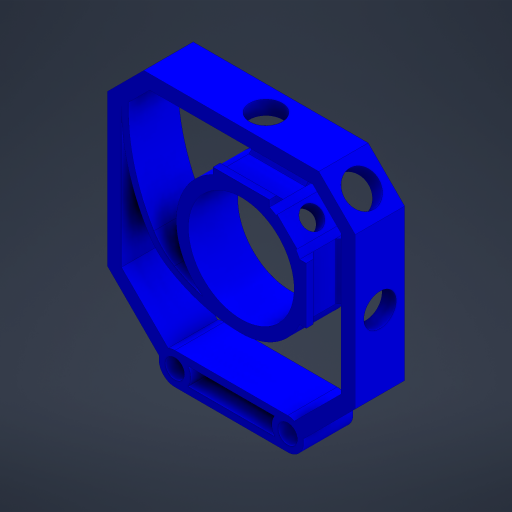
# Autodesk Inventor part: Laser Holder (Green Laser)
Saved by Autodesk Inventor 2023.4 (Build 274418000, 418)
## iProperties
Created: 2022-07-25
Part Number: Laser Holder (Green Laser)
Material: Generic
Document SubType Name: Modeling
Designer: xSibe
Density: 1 g/cm^3
Appearance: Plastic Blue
Author: xSibe
Autodesk Inventor part; units mm, degrees
ref_plane "YZ Plane" through (0, 0, 0) normal (1, 0, 0) x (0, 1, 0)
ref_plane "XZ Plane" through (0, 0, 0) normal (0, 1, 0) x (-1, 0, 0)
ref_plane "XY Plane" through (0, 0, 0) normal (0, 0, 1) x (1, 0, 0)
sketch "Sketch1" plane through (0, 0, 0) normal (0, 0, 1) x (1, 0, 0)
  circle A0 centre (10, 3.85) radius 1.5625
  circle A1 centre (-10, 3.85) radius 1.5625
  line L0 (-16.9, 0) -> (16.9, 0)
  line L1 (16.9, 0) -> (16.9, 7.7)
  line L2 (-16.9, 7.7) -> (16.9, 7.7)
  line L3 (-16.9, 0) -> (-16.9, 7.7)
  circle A2 centre (-10, 3.85) radius 2.8125
  circle A3 centre (10, 3.85) radius 2.8125
  line L4 (-10, 6.6625) -> (10, 6.6625)
  line L5 (10, 1.0375) -> (-10, 1.0375)
  line L6 (-10, 2.2875) -> (10, 2.2875)
  line L7 (-10, 5.4125) -> (10, 5.4125)
  line L8 (-17.05, 7.7) -> (-17.05, 42.1)
  line L9 (17.05, 7.7) -> (17.05, 42.1)
  line L10 (-17.05, 24.9) -> (17.05, 24.9)
  line L11 (0, 24.9) -> (1.767767, 26.667767)
  line L12 (0, 24.9) -> (2.5, 24.9) construction
  circle A4 centre (1.767767, 26.667767) radius 9.375
  circle A5 centre (1.767767, 26.667767) radius 6.875
  circle A6 centre (1.767767, 26.667767) radius 11.5
  line L13 (1.767767, 26.667767) -> (1.767767, 38.167767)
  line L14 (1.767767, 38.167767) -> (1.767767, 37.542767)
  line L15 (-3.232233, 36.917767) -> (6.767767, 36.917767)
  line L16 (6.767767, 36.917767) -> (6.767767, 38.167767)
  line L17 (6.767767, 38.167767) -> (-3.232233, 38.167767)
  line L18 (-3.232233, 38.167767) -> (-3.232233, 36.917767)
  line L19 (-3.232233, 36.917767) -> (6.767767, 38.167767) construction
  line L20 (6.767767, 36.917767) -> (-3.232233, 38.167767) construction
  line L21 (1.767767, 26.667767) -> (9.899495, 34.799495)
  line L22 (9.899495, 34.799495) -> (9.457553, 34.357553)
  line L23 (11.667262, 33.031728) -> (8.131728, 36.567262)
  line L24 (8.131728, 36.567262) -> (7.247845, 35.683378)
  line L25 (7.247845, 35.683378) -> (10.783378, 32.147845)
  line L26 (10.783378, 32.147845) -> (11.667262, 33.031728)
  line L27 (11.667262, 33.031728) -> (7.247845, 35.683378) construction
  line L28 (8.131728, 36.567262) -> (10.783378, 32.147845) construction
  line L29 (11.667262, 33.031728) -> (16.667262, 33.031728) construction
  line L30 (12.017767, 21.667767) -> (12.017767, 31.667767)
  line L31 (12.017767, 31.667767) -> (13.267767, 31.667767)
  line L32 (13.267767, 31.667767) -> (13.267767, 21.667767)
  line L33 (13.267767, 21.667767) -> (12.017767, 21.667767)
  line L34 (1.767767, 38.167767) -> (1.767767, 40.167767)
  line L35 (13.267767, 26.667767) -> (15.267767, 26.667767)
  line L36 (-10.217767, 5.432233) -> (10.217767, 5.432233)
  line L37 (19.467767, 14.682233) -> (19.467767, 39.367767)
  line L38 (14.467767, 44.367767) -> (-14.467767, 44.367767)
  line L39 (-19.467767, 39.367767) -> (-19.467767, 14.682233)
  line L40 (-19.467767, 5.432233) -> (19.467767, 44.367767) construction
  line L41 (19.467767, 5.432233) -> (-19.467767, 44.367767) construction
  line L42 (-10.217767, 5.432233) -> (-19.467767, 14.682233)
  line L43 (10.217767, 5.432233) -> (19.467767, 14.682233)
  line L44 (14.467767, 44.367767) -> (19.467767, 39.367767)
  line L45 (-14.467767, 44.367767) -> (-19.467767, 39.367767)
  line L46 (-15.503301, 46.867767) -> (-21.967767, 40.403301)
  line L47 (-21.967767, 40.403301) -> (-21.967767, 13.646699)
  line L48 (-21.967767, 13.646699) -> (-11.253301, 2.932233)
  line L49 (-11.253301, 2.932233) -> (11.253301, 2.932233)
  line L50 (11.253301, 2.932233) -> (21.967767, 13.646699)
  line L51 (21.967767, 13.646699) -> (21.967767, 40.403301)
  line L52 (21.967767, 40.403301) -> (15.503301, 46.867767)
  line L53 (15.503301, 46.867767) -> (-15.503301, 46.867767)
  circle A7 centre (-10, 3.85) radius 1.705
  circle A8 centre (10, 3.85) radius 1.707
  line L54 (1.767767, 15.167767) -> (-13.232233, 15.167767)
  line L55 (-13.232233, 15.167767) -> (-13.232233, 20.167767)
  arc A9 (-19.467767, 39.367767) -> (-13.232233, 20.167767) centre (13.209618, 39.367767) ccw
  arc A10 (-13.232233, 20.167767) -> (1.767767, 15.167767) centre (1.767767, 40.167767) ccw
  arc A11 (-18.191856, 40.643678) -> (-12.331418, 21.055586) centre (13.209618, 39.367767) ccw
  arc A12 (-12.331418, 21.055586) -> (-5.074449, 17.424711) centre (1.767767, 40.167767) ccw
  line L56 (-12.331418, 21.055586) -> (-13.70616, 23.143667)
  line L57 (-13.232233, 20.167767) -> (-14.62268, 22.245423)
  arc A13 (-13.70616, 23.143667) -> (-10.054119, 19.56909) centre (-4.985941, 28.399978) ccw
  arc A14 (-14.62268, 22.245423) -> (-10.979773, 18.661949) centre (-5.545684, 27.829564) ccw
  point P0 (0, 0)
  point P1 (-7.661464, 2.2875)
  point P2 (-7.661464, 5.4125)
  point P3 (7.661464, 5.4125)
  point P4 (7.661464, 2.2875)
  point P5 (7.341455, 2.932233)
  point P6 (-7.341455, 2.932233)
  point P7 (-11.185824, 6.40029)
  point P8 (11.185824, 6.40029)
  point P9 (-3.232233, 37.023925)
  point P10 (12.123925, 21.667767)
  point P11 (12.123925, 31.667767)
  point P12 (11.472788, 32.837254)
  point P13 (7.937254, 36.372788)
  point P14 (6.767767, 37.023925)
  point P15 (12.751875, 4.430808)
  point P16 (-12.751875, 4.430808)
  dimension "d0" = 1.25
  dimension "d1" = 1.25
  dimension "d2" = 2.5
  dimension "d3" = 45
  dimension "d4" = 18.75
  dimension "d5" = 2.5
  dimension "d6" = 2.125
  dimension "d7" = 0.625
  dimension "d8" = 10
  dimension "d9" = 1.25
  dimension "d10" = 0.625
  dimension "d11" = 5
  dimension "d12" = 135
  dimension "d13" = 1.25
  dimension "d14" = 2
  dimension "d15" = 2
  dimension "d16" = 38.93553
  dimension "d17" = 38.93553
  dimension "d18" = 9.25
  dimension "d19" = 9.25
  dimension "d20" = 9.25
  dimension "d21" = 9.25
  dimension "d22" = 5
  dimension "d23" = 5
  dimension "d24" = 5
  dimension "d25" = 5
  dimension "d26" = 2.5
  dimension "d46" = 0.1425
  dimension "d47" = 0.1445
  dimension "d48" = 15
  dimension "d49" = 5
  dimension "d50" = 1.25
  dimension "d51" = 2.5
  dimension "d52" = 2.5
  constraints: 104 end point, 28 point on circle, 14 tangent, 13 centre point, 12 point on line, 10 midpoint, 8 parallel, 7 horizontal, 7 perpendicular, 4 symmetric about line, 2 equal length, 1 coincident, 1 vertical, 8 other
  measures "d0" radial gap between concentric circles of A1 A2
  measures "d1" radial gap between concentric circles of A0 A3
  measures "d2" distance of L11.start L11.end
  measures "d3" angle of L12 L11
  measures "d4" diameter of A4
  measures "d5" radial gap between concentric circles of A4 A5
  measures "d6" radial gap between concentric circles of A4 A6
  measures "d7" distance of L13.end L14.end
  measures "d8" distance of L17.end L16.end
  measures "d9" distance of L16.end L15.end
  measures "d10" distance of L21.end L22.end
  measures "d11" distance of L23.start L23.end
  measures "d12" angle of L29 L23
  measures "d13" distance of L24.end L23.end
  measures "d14" distance of L13.end L34.end
  measures "d15" distance of L35.start L35.end
  measures "d16" distance of L40.end L41.end
  measures "d17" distance of L41.end L40.start
  measures "d18" distance of L36.start L40.start
  measures "d19" distance of L39.end L40.start
  measures "d20" distance of L36.end L41.start
  measures "d21" distance of L37.start L41.start
  measures "d22" distance of L38.start L40.end
  measures "d23" distance of L37.end L40.end
  measures "d24" distance of L38.end L41.end
  measures "d25" distance of L39.start L41.end
  measures "d26" distance between parallel lines of L38 L53
  measures "d46" radial gap between concentric circles of A1 A7
  measures "d47" radial gap between concentric circles of A0 A8
  measures "d48" distance of L54.start L54.end
  measures "d49" distance of L54.end L55.end
  measures "d50" radial gap between concentric circles of A9 A11
  measures "d51" distance of L56.start L56.end
  measures "d52" distance of L55.end L57.end
extrude "Extrusion1" add sketch "Sketch1" along normal mid plane 8.75 contours A8 L49 A3 L7 | L7 A3 L36 A8 | A8 L43 A3 L50 | L50 A3 L6 A8 | A8 L6 A3 L49 | L7 A2 L36 A3 | L36 A3 L43 A8 | A3 L43 L2 L50 | L36 A2 L4 A3 | L7 A7 L36 A2 | A2 L49 A7 L7 | A3 L5 A2 L6 | L2 L43 L9 L50 | A2 L6 A7 L49 | L36 A7 L42 A2 | A2 L48 A7 L6 | L9 L43 L37 L44 L38 L45 L39 L42 L8 L48 L47 L46 L53 L52 L51 L50 | L42 A2 L48 L2 | L2 L48 L8 L42 | L42 A7 L48 A2 | L32 L33 A6 L10 | L10 A6 L32 | A9 L45 A11 L8 | L8 A11 L10 A9 | L10 A11 A12 A6 A10 A14 L57 A9 | A6 L33 L30 L10 | L10 L30 L31 A6 | A6 L31 L32 | L57 A14 | L30 L33 A6 L10 A4 | L10 A4 L21 L25 L26 A6 L31 L30 | A6 L18 L15 L13 A4 L10 | A13 L56 A11 | L26 L25 L21 A6 | A6 L23 L26 | L18 L17 A6 | A6 L13 L15 L18 | L56 A13 A12 | L21 L25 L24 A6 | A6 L24 L23 | L13 L15 L16 A6 L24 L25 L21 A4 | L17 L16 A6 | A6 L16 L15 L13
sketch "Sketch2" plane through (0, 0, 0) normal (0, 0, 1) x (1, 0, 0)
  circle A0 centre (1.767767, 26.667767) radius 9.375
  circle A1 centre (1.767767, 26.667767) radius 7.5
  point P0 (0, 0)
  dimension "d30" = 1.875
  constraints: 1 centre point
  measures "d30" radial gap between concentric circles of A0 A1
extrude "Extrusion2" [suppressed]
sketch "Sketch3" plane through (21.967767, 13.646699, -4.375) normal (1, 0, 0) x (0, 0, -1)
  line L0 (0, 8.021068) -> (-8.75, 8.021068)
  line L1 (0, 18.021068) -> (0, 8.021068)
  line L2 (0, 18.021068) -> (-8.75, 18.021068)
  line L3 (-8.75, 8.021068) -> (-8.75, 18.021068)
  line L4 (-4.375, 18.021068) -> (-4.375, 8.021068)
  circle A0 centre (-4.375, 13.021068) radius 2.875
  point P0 (-4.375, -13.646699)
  dimension "d33" = 5.75
  constraints: 3 midpoint, 2 end point, 1 centre point
  measures "d33" diameter of A0
extrude "Extrusion3" cut sketch "Sketch3" against normal up to surface (2.5 mm away) contours A0 L4 | L4 A0
sketch "Sketch4" plane through (12.123925, 31.667767, -4.375) normal (0, 1, 0) x (1, 0, 0)
  line L0 (1.143842, 0) -> (1.143842, -8.75)
  line L1 (0, 0) -> (1.143842, 0)
  line L2 (0, 0) -> (0, -8.75)
  line L3 (1.143842, -8.75) -> (0, -8.75)
  line L4 (1.143842, -8.75) -> (0, -8.75)
  line L5 (0, -8.75) -> (0, -7.5)
  line L6 (0, -7.5) -> (1.143842, -7.5)
  line L7 (1.143842, -7.5) -> (1.143842, -8.75)
  line L8 (1.143842, -7.5) -> (0, -6.356158)
  line L9 (1.143842, -7.5) -> (2.76148, -7.5) construction
  line L10 (0, -4.375) -> (1.143842, -4.375)
  line L11 (1.143842, -1.25) -> (0, -2.393842)
  point P0 (-12.123925, -4.375)
  point P1 (1.143842, -1.25)
  point P2 (0, -2.393842)
  point P3 (1.143842, -7.5)
  dimension "d36" = 1.25
  dimension "d37" = 135
  constraints: 16 end point, 2 horizontal, 2 midpoint, 2 parallel, 2 point on line, 2 symmetric about line, 1 equal length, 1 perpendicular
  measures "d36" distance of L4.end L5.end
  measures "d37" angle of L9 L8
extrude "Extrusion4" cut sketch "Sketch4" against normal up to surface (10 mm away) contours L0 L10 L2 L11 | L0 L8 L2 L10
ref_plane "Work Plane1" through (13.267767, 38.167767, 4.375) normal (0.7071068, -0.7071068, 0) x (0, 0, -1)
mirror "Mirror1" about plane through (13.267767, 38.167767, 4.375) normal (0.7071068, -0.7071068, 0) of "Extrusion3", "Extrusion4"
sketch "Sketch5" plane through (21.967767, 40.403301, 4.375) normal (0.7071068, 0.7071068, 0) x (0.7071068, -0.7071068, 0)
  line L0 (0, 8.75) -> (0, 0)
  line L1 (-9.142136, 8.75) -> (0, 8.75)
  line L2 (-9.142136, 8.75) -> (-9.142136, 0)
  line L3 (0, 0) -> (-9.142136, 0)
  line L4 (-2.071068, 8.75) -> (-2.071068, 0)
  line L5 (-7.071068, 8.75) -> (-2.071068, 8.75)
  line L6 (-7.071068, 8.75) -> (-7.071068, 0)
  line L7 (-2.071068, 0) -> (-7.071068, 0)
  circle A0 centre (-4.571068, 4.375) radius 1.875
  line L8 (-7.071068, 4.375) -> (-2.071068, 4.375)
  circle A1 centre (-4.571068, 4.375) radius 3
  point P0 (13.035891, 4.375)
  dimension "d40" = 3.75
  dimension "d41" = 6
  constraints: 3 midpoint, 2 centre point, 2 end point, 1 coincident
  measures "d40" diameter of A0
  measures "d41" diameter of A1
extrude "Extrusion5" cut sketch "Sketch5" against normal up to surface (2.5 mm away) contours A1 L4 | L4 L8 A0 L6 A1 | A1 L6 L8 A0 L4 | L6 A1 | L8 A0 | A0 L8
extrude "Extrusion6" cut sketch "Sketch5" against normal up to surface from surface at -12.496046 contours L8 A0 | A0 L8 round surface about axis through (1.767767, 26.667767, 0) along (0, 0, 1) radius 9.375 far side no
equation "\"d19\" = d18"
equation "\"d20\" = d18"
equation "\"d21\" = d20"
equation "\"d23\" = d22"
equation "\"d24\" = d22"
equation "\"d25\" = d24"
body "Solid1"
